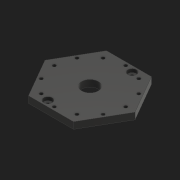
# Autodesk Inventor part: AC04
Saved by Autodesk Inventor 2017 (Build 210142000, 142)
## iProperties
Created: 2019-08-28
Part Number: AC04
Material: ABS Plastic
Document SubType Name: Modeling
Designer: Dell
Density: 1.06 g/cm^3
Appearance: Smooth - Black
Author: Dell
Autodesk Inventor part; units mm, degrees
ref_plane "YZ Plane" through (0, 0, 0) normal (1, 0, 0) x (0, 1, 0)
ref_plane "XZ Plane" through (0, 0, 0) normal (0, 1, 0) x (-1, 0, 0)
ref_plane "XY Plane" through (0, 0, 0) normal (0, 0, 1) x (1, 0, 0)
sketch "Sketch1" plane through (0, 0, 0) normal (0, 0, 1) x (1, 0, 0)
  line L0 (77.9423, 0) -> (38.9711, -67.5)
  line L1 (38.9711, -67.5) -> (-38.9711, -67.5)
  line L2 (-38.9711, -67.5) -> (-77.9423, 0)
  line L3 (-77.9423, 0) -> (-38.9711, 67.5)
  line L4 (-38.9711, 67.5) -> (38.9711, 67.5)
  line L5 (38.9711, 67.5) -> (77.9423, 0)
  circle A0 centre (0, 0) radius 12.5
  circle A1 centre (54, 0) radius 2.5
  circle A2 centre (46.7654, 27) radius 2.5
  circle A3 centre (27, 46.7654) radius 2.5
  circle A4 centre (0, 54) radius 2.5
  circle A5 centre (-27, 46.7654) radius 2.5
  circle A6 centre (-46.7654, 27) radius 2.5
  circle A7 centre (-54, 0) radius 2.5
  circle A8 centre (-46.7654, -27) radius 2.5
  circle A9 centre (-27, -46.7654) radius 2.5
  circle A10 centre (0, -54) radius 2.5
  circle A11 centre (27, -46.7654) radius 2.5
  circle A12 centre (46.7654, -27) radius 2.5
  dimension "d0" = 135
  dimension "d1" = 25
  dimension "d2" = 54
  dimension "d3" = 5
  dimension "d6" = 360
  constraints: 13 centre point, 12 end point, 2 coincident, 2 horizontal alignment, 38 other
  measures "d0" distance between parallel lines of L1 L4
  measures "d1" diameter of A0
  measures "d2" distance of A1.centre point (0, 0)
  measures "d3" diameter of A1
extrude "Extrusion1" add sketch "Sketch1" along normal blind 10
sketch "Sketch5" plane through (0, 0, 10) normal (0, 0, 1) x (1, 0, 0)
  circle A0 centre (0, 0) radius 12.5 projected
  circle A1 centre (46.7654, -27) radius 2.5 projected
  circle A2 centre (27, -46.7654) radius 2.5 projected
  circle A3 centre (-27, -46.7654) radius 2.5 projected
  circle A4 centre (-46.7654, -27) radius 2.5 projected
  circle A5 centre (-54, 0) radius 2.5 projected
  circle A6 centre (-46.7654, 27) radius 2.5 projected
  circle A7 centre (-27, 46.7654) radius 2.5 projected
  circle A8 centre (27, 46.7654) radius 2.5 projected
  circle A9 centre (46.7654, 27) radius 2.5 projected
  circle A10 centre (54, 0) radius 2.5 projected
  line L0 (38.9711, -67.5) -> (77.9423, 0) projected
  line L1 (77.9423, 0) -> (38.9711, 67.5) projected
  line L2 (38.9711, 67.5) -> (-38.9711, 67.5) projected
  line L3 (-38.9711, 67.5) -> (-77.9423, 0) projected
  line L4 (-77.9423, 0) -> (-38.9711, -67.5) projected
  line L5 (-38.9711, -67.5) -> (38.9711, -67.5) projected
  line L6 (-68.1273, 0) -> (-34.0637, 59)
  line L7 (-34.0637, 59) -> (34.0637, 59)
  line L8 (34.0637, 59) -> (68.1273, 0)
  line L9 (68.1273, 0) -> (34.0637, -59)
  line L10 (34.0637, -59) -> (-34.0637, -59)
  line L11 (-34.0637, -59) -> (-68.1273, 0)
  dimension "d30" = 118
  constraints: 12 end point, 5 other
  measures "d30" distance between parallel lines of L9 L6
extrude "Extrusion5" cut sketch "Sketch5" against normal through all contours L5 L4 L3 L2 L1 L0
sketch "Sketch6" plane through (0, 0, 10) normal (0, 0, 1) x (1, 0, 0)
  circle A0 centre (0, 52) radius 2.5
  circle A1 centre (-13.4586, 50.2281) radius 2.5
  circle A2 centre (-26, 45.0333) radius 2.5
  circle A3 centre (-36.7696, 36.7696) radius 2.5
  circle A4 centre (-45.0333, 26) radius 2.5
  circle A5 centre (-50.2281, 13.4586) radius 2.5
  circle A6 centre (-52, 0) radius 2.5
  circle A7 centre (-50.2281, -13.4586) radius 2.5
  circle A8 centre (-45.0333, -26) radius 2.5
  circle A9 centre (-36.7696, -36.7696) radius 2.5
  circle A10 centre (-26, -45.0333) radius 2.5
  circle A11 centre (-13.4586, -50.2281) radius 2.5
  circle A12 centre (0, -52) radius 2.5
  circle A13 centre (13.4586, -50.2281) radius 2.5
  circle A14 centre (26, -45.0333) radius 2.5
  circle A15 centre (36.7696, -36.7696) radius 2.5
  circle A16 centre (45.0333, -26) radius 2.5
  circle A17 centre (50.2281, -13.4586) radius 2.5
  circle A18 centre (52, 0) radius 2.5
  circle A19 centre (50.2281, 13.4586) radius 2.5
  circle A20 centre (45.0333, 26) radius 2.5
  circle A21 centre (36.7696, 36.7696) radius 2.5
  circle A22 centre (26, 45.0333) radius 2.5
  circle A23 centre (13.4586, 50.2281) radius 2.5
  point P0 (0, 0)
  dimension "d35" = 5
  dimension "d38" = 360
  dimension "d40" = 52
  constraints: 24 centre point, 1 vertical alignment, 49 other
  measures "d35" diameter of A0
  measures "d40" distance of point (0, 0) A0.centre
extrude "Extrusion6" cut sketch "Sketch6" against normal through all contours A11 | A23
sketch "Sketch7" plane through (0, 0, 10) normal (0, 0, 1) x (1, 0, 0)
  circle A0 centre (13.4586, 50.2281) radius 2.5 projected
  circle A1 centre (-13.4586, -50.2281) radius 2.5 projected
  circle A2 centre (13.4586, 50.2281) radius 6.5
  circle A3 centre (-13.4586, -50.2281) radius 6.5
  point P0 (0, 0)
  dimension "d43" = 13
  dimension "d44" = 13
  constraints: 2 centre point, 2 coincident
  measures "d43" diameter of A2
  measures "d44" diameter of A3
extrude "Extrusion7" cut sketch "Sketch7" against normal blind 5 contours A0 | A1 | A2 | A3
body "Solid1"
